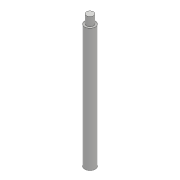
# Autodesk Inventor part: 車軸
Saved by Autodesk Inventor 2017 (Build 210142000, 142)
## iProperties
Part Number: 車軸
Material: 一般
Document SubType Name: Modeling
Designer: highs
Density: 1 g/cm^3
Appearance: 既定
Author: highs
Autodesk Inventor part; units mm, degrees
ref_plane "YZ Plane" through (0, 0, 0) normal (1, 0, 0) x (0, 1, 0)
ref_plane "XZ Plane" through (0, 0, 0) normal (0, 1, 0) x (-1, 0, 0)
ref_plane "XY Plane" through (0, 0, 0) normal (0, 0, 1) x (1, 0, 0)
sketch "スケッチ1" plane through (0, 0, 0) normal (0, 0, 1) x (1, 0, 0)
  line L0 (0, 0) -> (0, -6) construction
  circle A0 centre (0, -6) radius 6
  dimension "d0" = 12
  constraints: 2 end point, 1 coincident, 1 vertical, 1 vertical alignment, 2 other
extrude "押し出し1" add sketch "スケッチ1" along normal blind 150
sketch "スケッチ4" plane through (0, -6, 150) normal (0, 0, 1) x (1, 0, 0)
  circle A0 centre (0, 0) radius 6
  circle A1 centre (0, 0) radius 4
  circle A2 centre (0, 0) radius 6 projected
  point P0 (0, 6)
  dimension "d9" = 8
  constraints: 2 centre point, 2 coincident, 1 vertical alignment, 1 other
  measures "d9" diameter of A1
extrude "押し出し3" cut sketch "スケッチ4" against normal blind 10
